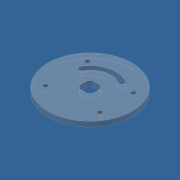
# Autodesk Inventor part: S1702_couverclehaut
Saved by Autodesk Inventor 2015 SP2 (Build 190223200, 223)
## iProperties
Created: 2017-10-31
Part Number: S1702_couverclehaut
Project: S1702_Circuit_Course
Material: Plastique PMMA
Description: Couvercle Haut
Document SubType Name: Modeling
Designer: Benoit.CURCHOD2
Authority: Ø50x3
Density: 1.188 g/cm^3
Appearance: Transparent - Clair
Mass: 6.45604 g
Surface Area: 44.316 cm^2
Volume: 5.43438 cm^3
Material number: ---
Author: Benoit.CURCHOD2
Autodesk Inventor part; units mm, degrees
ref_plane "Plan YZ" through (0, 0, 0) normal (1, 0, 0) x (0, 1, 0)
ref_plane "Plan XZ" through (0, 0, 0) normal (0, 1, 0) x (-1, 0, 0)
ref_plane "Plan XY" through (0, 0, 0) normal (0, 0, 1) x (1, 0, 0)
sketch "Esquisse1" plane through (0, 0, 0) normal (0, 0, 1) x (1, 0, 0)
  circle A0 centre (0, 0) radius 25
  dimension "d0" = 50
  constraints: 1 centre point, 1 coincident
  measures "d0" diameter of A0
extrude "Extrusion1" add sketch "Esquisse1" along normal blind 3
sketch "Esquisse6" plane through (0, 0, 3) normal (0, 0, 1) x (1, 0, 0)
  circle A0 centre (0, 0) radius 14 construction
  line L0 (-48.7218, 0) -> (37.287, 0) construction
  line L1 (0, -36.4494) -> (0, 43.6964) construction
  line L2 (0, 0) -> (-36.4348, 21.0356) construction
  line L3 (0, 0) -> (18.6178, 32.247) construction
  arc A1 (7.75, 13.4234) -> (-13.4234, 7.75) centre (0, 0) ccw
  arc A2 (6.25, 10.8253) -> (-10.8253, 6.25) centre (0, 0) ccw
  arc A3 (-13.4234, 7.75) -> (-10.8253, 6.25) centre (-12.1244, 7) ccw
  arc A4 (6.25, 10.8253) -> (7.75, 13.4234) centre (7, 12.1244) ccw
  dimension "d3" = 28
  dimension "d4" = 30
  dimension "d5" = 90
  dimension "d6" = 1.5
  dimension "d7" = 1.5
  constraints: 8 point on circle, 5 centre point, 4 end point, 4 point on line, 4 tangent, 2 concentric, 1 coincident
  measures "d3" diameter of A0
  measures "d4" angle of L2 L0
  measures "d5" angle of L3 L2
  measures "d6" radial gap between concentric circles of A0 A1
  measures "d7" radial gap between concentric circles of A2 A0
extrude "Extrusion2" cut sketch "Esquisse6" against normal through all
sketch "Esquisse7" plane through (0, 0, 3) normal (0, 0, 1) x (1, 0, 0)
  circle A0 centre (0, 0) radius 4.6 construction
  line L0 (-35, 0) -> (35, 0) construction
  line L1 (0, -35) -> (0, 35) construction
  line L2 (-4.05, -4.05) -> (4.05, -4.05) construction
  line L3 (4.05, -4.05) -> (4.05, 4.05) construction
  line L4 (4.05, 4.05) -> (-4.05, 4.05) construction
  line L5 (-4.05, 4.05) -> (-4.05, -4.05) construction
  line L6 (0, -4.05) -> (-2.1812, -4.05)
  line L7 (-4.05, -2.1812) -> (-4.05, 0)
  arc A1 (-4.05, -2.1812) -> (-2.1812, -4.05) centre (0, 0) ccw
  line L8 (0, 4.05) -> (-2.1812, 4.05)
  line L9 (-4.05, 2.1812) -> (-4.05, 0)
  arc A2 (-2.1812, 4.05) -> (-4.05, 2.1812) centre (0, 0) ccw
  line L10 (0, -4.05) -> (2.1812, -4.05)
  line L11 (4.05, -2.1812) -> (4.05, 0)
  arc A3 (2.1812, -4.05) -> (4.05, -2.1812) centre (0, 0) ccw
  line L12 (4.05, 2.1812) -> (4.05, 0)
  arc A4 (4.05, 2.1812) -> (2.1812, 4.05) centre (0, 0) ccw
  line L13 (0, 4.05) -> (2.1812, 4.05)
  dimension "d10" = 9.2
  dimension "d13" = 8.1
  constraints: 24 end point, 10 point on circle, 8 symmetric about line, 5 centre point, 4 midpoint, 2 parallel, 2 perpendicular, 2 point on line, 1 coincident, 1 concentric, 1 horizontal, 5 other
  measures "d10" diameter of A0
  measures "d13" distance between parallel lines of L4 L2
extrude "Extrusion3" cut sketch "Esquisse7" against normal through all
sketch "Esquisse8" plane through (0, 0, 3) normal (0, 0, 1) x (1, 0, 0)
  circle A0 centre (0, 0) radius 18.8 construction
  line L0 (-35, 0) -> (35, 0) construction
  point P0 (-14.0424, 12.5)
  point P1 (-14.0424, -12.5)
  point P2 (15.9198, 10)
  point P3 (15.9198, -10)
  dimension "d16" = 37.6
  dimension "d25" = 25
  dimension "d26" = 20
  constraints: 4 point on circle, 2 symmetric about line, 1 centre point, 1 coincident
  measures "d16" diameter of A0
  measures "d25" distance of A0.end A0.start
  measures "d26" distance of point (15.92, -10) point (15.92, 10)
hole "Perçage1" at (-14.0424, -12.5, 3) at (-14.0424, 12.5, 3) at (15.9198, 10, 3) at (15.9198, -10, 3) direction (0, 0, -1) diameter 2.459 depth 8.5 tip angle 118 thread size "M3x0.5" class "6H" standard "ISO M"
